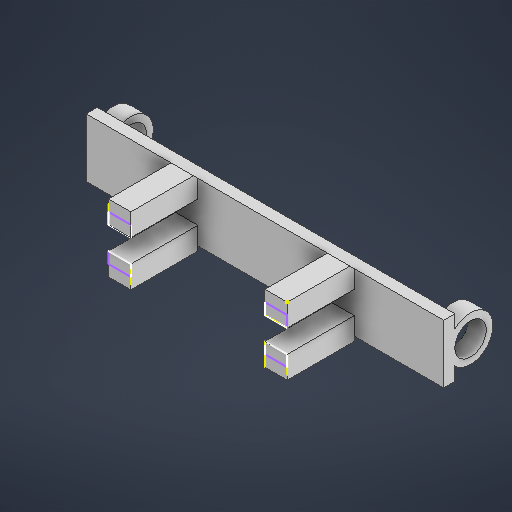
# Autodesk Inventor part: sccop_mount
Saved by Autodesk Inventor 2026.1 (Build 301233020, 233B)
## iProperties
Created: 2026-02-04
Part Number: sccop_mount
Material: Generic
Document SubType Name: Modeling
Designer: Dylan
Density: 1 g/cm^3
Appearance: Default
Author: Dylan
Autodesk Inventor part; units mm, degrees
ref_plane "YZ Plane" through (0, 0, 0) normal (1, 0, 0) x (0, 1, 0)
ref_plane "XZ Plane" through (0, 0, 0) normal (0, 1, 0) x (-1, 0, 0)
ref_plane "XY Plane" through (0, 0, 0) normal (0, 0, 1) x (1, 0, 0)
sketch "Sketch1" plane through (0, 0, 0) normal (0, 0, 1) x (1, 0, 0)
  line L0 (0, 0) -> (-5, 0)
  line L1 (-5, 0) -> (-5, -5)
  line L2 (-5, -5) -> (0, -5)
  line L3 (0, -5) -> (0, 0)
  line L4 (-40, 0) -> (-35, 0)
  line L5 (-35, 0) -> (-35, -5)
  line L6 (-35, -5) -> (-40, -5)
  line L7 (-40, -5) -> (-40, 0)
  line L8 (0, -15.1) -> (-5, -15.1)
  line L9 (-5, -15.1) -> (-5, -10.1)
  line L10 (-5, -10.1) -> (0, -10.1)
  line L11 (0, -10.1) -> (0, -15.1)
  line L12 (-40, -15.1) -> (-35, -15.1)
  line L13 (-35, -15.1) -> (-35, -10.1)
  line L14 (-35, -10.1) -> (-40, -10.1)
  line L15 (-40, -10.1) -> (-40, -15.1)
  line L16 (0, 0) -> (-5, 0)
  line L17 (-35, 0) -> (-40, 0)
  line L18 (0, -15.1) -> (0, -10.1)
  line L19 (0, -5) -> (0, 0)
  line L20 (-40, -15.1) -> (-35, -15.1)
  line L21 (-5, -15.1) -> (0, -15.1)
  line L22 (-40, 0) -> (-40, -5)
  line L23 (-40, -10.1) -> (-40, -15.1)
  dimension "d0" = 40
  dimension "d1" = 15.1
  dimension "d2" = 5
  dimension "d3" = 5
  dimension "d4" = 5
  dimension "d5" = 5
  dimension "d6" = 5
  dimension "d7" = 5
  dimension "d8" = 5
  dimension "d9" = 5
  constraints: 48 end point, 16 parallel, 8 perpendicular, 6 horizontal
  measures "d0" distance of L8.start L12.start
  measures "d1" distance of L12.start L4.start
  measures "d2" distance of L2.end L1.end
  measures "d3" distance of L1.end L0.end
  measures "d4" distance of L5.end L6.end
  measures "d5" distance of L4.end L5.end
  measures "d6" distance of L9.end L10.end
  measures "d7" distance of L8.end L9.end
  measures "d8" distance of L14.end L13.end
  measures "d9" distance of L13.end L12.end
extrude "Mounting arms" add sketch "Sketch1" along normal blind 15
sketch "Sketch2" plane through (0, 0, 0) normal (0, 0, -1) x (-1, 0, 0)
  line L0 (-19.9999, -1.0001) -> (59.9998, -1.0001)
  line L1 (59.9998, -1.0001) -> (59.9998, -14.0997)
  line L2 (59.9998, -14.0997) -> (-19.9999, -14.0997)
  line L3 (-19.9999, -14.0997) -> (-19.9999, -1.0001)
  point P0 (0, 0)
  constraints: 8 end point, 2 parallel, 1 horizontal, 1 perpendicular
extrude "Plate" add sketch "Sketch2" along normal blind 2.5
sketch "Sketch3" plane through (19.9999, -14.0997, 0) normal (1, 0, 0) x (0, 0, -1)
  circle A0 centre (6, 6.5498) radius 5
  point P0 (0, 14.0997)
  dimension "d14" = 10
  constraints: 1 centre point
  measures "d14" diameter of A0
sketch "Sketch5" plane through (-59.9998, -14.0997, 0) normal (-1, 0, 0) x (0, 0, 1)
  circle A0 centre (-6, 6.5498) radius 5
  point P0 (0, 14.0997)
  dimension "d15" = 10
  constraints: 1 centre point
  measures "d15" diameter of A0
extrude "retainer1" add sketch "Sketch5" against normal blind 4
extrude "retainer2" add sketch "Sketch3" against normal blind 4
sketch "Sketch6" plane through (-59.9998, -14.0997, 0) normal (-1, 0, 0) x (0, 0, 1)
  line L0 (0, 13.0996) -> (0, 0) projected
  circle A0 centre (-5.9997, 6.4943) radius 3.5
  point P0 (0, 14.0997)
  dimension "d21" = 7
  constraints: 1 centre point
  measures "d21" diameter of A0
extrude "cyldiner shaft holes" cut sketch "Sketch6" against normal blind 80
chamfer "Chamfer1" distance 1 angle 45 2 edges at (-37.5, 0, 0) (-2.5, 0, 0)
sketch "Sketch7" plane through (0, 0, 15) normal (0, 0, 1) x (1, 0, 0)
  line L0 (-40, -1.0001) -> (-40, -5) projected
  line L1 (0, -14.0997) -> (0, -10.1) projected
  line L2 (-35, -14.0997) -> (-35, -10.1) projected
  line L3 (-40, -12.6005) -> (-35, -12.6005)
  line L4 (-35, -12.6005) -> (-35, -10.1)
  line L5 (-35, -10.1) -> (-40, -10.1)
  line L6 (-40, -10.1) -> (-40, -12.6005)
  line L7 (-5, -10.1) -> (-5, -15.1) projected
  line L8 (0, -12.6005) -> (-5, -12.6005)
  line L9 (-5, -12.6005) -> (-5, -10.1)
  line L10 (-5, -10.1) -> (0, -10.1)
  line L11 (0, -10.1) -> (0, -12.6005)
  line L12 (-5, -5) -> (0, -5) projected
  line L13 (0, -2.5001) -> (-5, -2.5001)
  line L14 (-5, -2.5001) -> (-5, -5)
  line L15 (-5, -5) -> (0, -5)
  line L16 (0, -5) -> (0, -2.5001)
  line L17 (-40, -2.5001) -> (-35, -2.5001)
  line L18 (-35, -2.5001) -> (-35, -5)
  line L19 (-35, -5) -> (-40, -5)
  line L20 (-40, -5) -> (-40, -2.5001)
  line L21 (-40, -2.5001) -> (-35, -2.5001)
  line L22 (-5, -2.5001) -> (0, -2.5001)
  line L23 (-40, -12.6005) -> (-40, -10.1)
  line L24 (-40, -5) -> (-40, -2.5001)
  line L25 (0, -12.6005) -> (-5, -12.6005)
  line L26 (-35, -12.6005) -> (-40, -12.6005)
  line L27 (0, -2.5001) -> (0, -5)
  line L28 (0, -10.1) -> (0, -12.6005)
  point P0 (0, 0)
  constraints: 48 end point, 16 parallel, 8 perpendicular, 6 horizontal, 4 point on line
body "Solid1"
